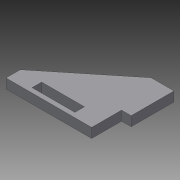
# Autodesk Inventor part: Mount_Mega_End
Saved by Autodesk Inventor 2014 (Build 180170000, 170)
## iProperties
Created: 2014-10-26
Part Number: Mount_Mega_End
Material: Generic
Document SubType Name: Modeling
Designer: ThatOtherGuy
Density: 1 g/cm^3
Appearance: Default
Author: ThatOtherGuy
Autodesk Inventor part; units mm, degrees
ref_plane "YZ Plane" through (0, 0, 0) normal (1, 0, 0) x (0, 1, 0)
ref_plane "XZ Plane" through (0, 0, 0) normal (0, 1, 0) x (-1, 0, 0)
ref_plane "XY Plane" through (0, 0, 0) normal (0, 0, 1) x (1, 0, 0)
sketch "Sketch1" plane through (0, 0, 0) normal (0, 0, 1) x (1, 0, 0)
  line L0 (0, 0) -> (43.269, 0)
  line L1 (43.269, 0) -> (43.269, 50)
  line L2 (43.269, 50) -> (50, 50)
  line L3 (50, 50) -> (50, 20)
  line L4 (50, 20) -> (43.269, 20)
  line L5 (43.269, 20) -> (43.269, 50)
  line L6 (3.269, 3.269) -> (23.269, 3.269)
  line L7 (23.269, 3.269) -> (23.269, 10)
  line L8 (23.269, 10) -> (3.269, 10)
  line L9 (3.269, 10) -> (3.269, 3.269)
  line L10 (0, 10) -> (3.269, 10)
  line L11 (23.269, 10) -> (43.269, 10)
  line L12 (43.269, 50) -> (40, 50)
  line L13 (0, 10) -> (0, 0)
  line L14 (0, 10) -> (0, 13.269)
  line L15 (0, 13.269) -> (40, 50)
  point P0 (13.269, 3.269)
  point P1 (13.269, 0)
  dimension "d2" = 30
  dimension "d3" = 20
  dimension "d5" = 6.731
  dimension "d6" = 10
  dimension "d9" = 3.269
  dimension "d11" = 20
  dimension "d12" = 20
  dimension "d14" = 3.269
  dimension "d15" = 3.269
  constraints: 32 end point, 6 perpendicular, 5 parallel, 3 horizontal, 2 collinear, 2 point on line, 1 coincident, 1 midpoint, 1 vertical alignment
  measures "d2" distance of L2.end L3.end
  measures "d3" distance of L7.end L8.end
  measures "d5" distance of L6.end L7.end
  measures "d6" distance between parallel lines of L0 L11
  measures "d9" distance between parallel lines of L9 L13
  measures "d11" distance between parallel lines of L1 L7
  measures "d12" distance between parallel lines of L0 L4
  measures "d14" distance of L10.start L14.end
  measures "d15" distance of L1.end L12.end
extrude "Extrusion1" add sketch "Sketch1" along normal blind 6.731 contours L13 L10 L9 L6 L7 L11 L1 L0 | L14 L15 L12 L1 L11 L8 L10 | L1 L2 L3 L4
fillet "Fillet1" radius 2 3 edges at (40, 50, 3.3655) (0, 13.269, 3.3655) (0, 0, 3.3655)
equation "\"d5\" = THICKB"
equation "\"d7\" = THICKB"
equation "\"THICKA\" = 3.175"
equation "\"THICKB\" = 6.731"
equation "\"THICKC\" = 12.7"
equation "\"THICKPLY\" = 5"
equation "\"MAGDIA\" = 9.5"
equation "\"BALLDIA\" = 12"
body "Solid1"
